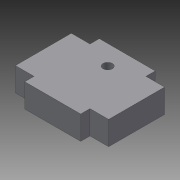
# Autodesk Inventor part: Air2D_Front_Feed
Saved by Autodesk Inventor 2014 (Build 180170000, 170)
## iProperties
Created: 2014-09-30
Part Number: Air2D_Front_Feed
Material: Generic
Document SubType Name: Modeling
Designer: ThatOtherGuy
Density: 1 g/cm^3
Appearance: Default
Author: ThatOtherGuy
Autodesk Inventor part; units mm, degrees
ref_plane "YZ Plane" through (0, 0, 0) normal (1, 0, 0) x (0, 1, 0)
ref_plane "XZ Plane" through (0, 0, 0) normal (0, 1, 0) x (-1, 0, 0)
ref_plane "XY Plane" through (0, 0, 0) normal (0, 0, 1) x (1, 0, 0)
sketch "Sketch1" plane through (0, 0, 0) normal (0, 0, 1) x (1, 0, 0)
  line L0 (-8.75, -10) -> (8.75, -10)
  line L1 (8.75, -10) -> (8.75, 10)
  line L2 (8.75, 10) -> (-8.75, 10)
  line L3 (-8.75, 10) -> (-8.75, -10)
  line L4 (8.75, 7.5) -> (13.75, 7.5)
  line L5 (13.75, 7.5) -> (13.75, -7.5)
  line L6 (13.75, -7.5) -> (8.75, -7.5)
  line L7 (8.75, -7.5) -> (8.75, 7.5)
  line L8 (-8.75, 7.5) -> (-13.75, 7.5)
  line L9 (-13.75, 7.5) -> (-13.75, -7.5)
  line L10 (-13.75, -7.5) -> (-8.75, -7.5)
  line L11 (-8.75, -7.5) -> (-8.75, 7.5)
  circle A0 centre (0, 4.75) radius 1.25
  point P0 (0, 0)
  point P1 (8.75, 0)
  point P2 (0, 10)
  point P3 (-13.75, 0)
  point P4 (13.75, 0)
  dimension "d0" = 5
  dimension "d1" = 17.5
  dimension "d2" = 20
  dimension "d3" = 15
  dimension "d7" = 8.75
  dimension "d9" = 2.5
  dimension "d10" = 2.5
  dimension "d11" = 4.75
  constraints: 24 end point, 6 parallel, 4 midpoint, 3 horizontal, 3 perpendicular, 2 equal length, 2 horizontal alignment, 2 point on line, 1 centre point, 1 vertical alignment
  measures "d0" distance of L8.start L8.end
  measures "d1" distance of L1.end L2.end
  measures "d2" distance of L2.end L0.start
  measures "d3" distance of L8.end L9.end
  measures "d7" distance from line of L1 A0.centre
  measures "d9" diameter of A0
  measures "d10" distance between parallel lines of L0 L6
  measures "d11" vertical distance of A0.centre point (-13.75, 0)
extrude "Extrusion1" add sketch "Sketch1" along normal blind 6.731
equation "\"d7\" = 0.5 * d1"
equation "\"d4\" = THICKB"
equation "\"THICKA\" = 3.175"
equation "\"THICKB\" = 6.731"
equation "\"THICKC\" = 12.7"
equation "\"BALLDIA\" = 12"
equation "\"MAGDIA\" = 9.5"
body "Solid1"
